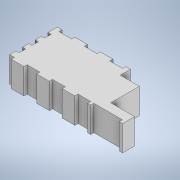
# Autodesk Inventor part: V9_BURROW_SIDE
Saved by Autodesk Inventor 2020.4 (Build 244396010, 396A)
## iProperties
Created: 2021-09-27
Part Number: V9_BURROW_SIDE
Material: Generic
Document SubType Name: Sheet Metal
Designer: YUSTE
Density: 1 g/cm^3
Sheet Metal Rule: Default
Appearance: Default
Author: YUSTE
Autodesk Inventor part; units mm, degrees
ref_plane "YZ Plane" through (0, 0, 0) normal (1, 0, 0) x (0, 1, 0)
ref_plane "XZ Plane" through (0, 0, 0) normal (0, 1, 0) x (-1, 0, 0)
ref_plane "XY Plane" through (0, 0, 0) normal (0, 0, 1) x (1, 0, 0)
sketch "Sketch1" plane through (0, 0, 0) normal (0, 1, 0) x (-1, 0, 0)
  line L0 (147.3507, -0.6443) -> (74.3257, -0.6443)
  line L1 (74.3257, -0.6443) -> (74.3257, 50.1557)
  line L2 (74.3257, 50.1557) -> (147.3507, 50.1557)
  line L3 (147.3507, 50.1557) -> (147.3507, -0.6443)
  line L4 (147.3507, 50.1557) -> (142.5882, 50.1557)
  line L5 (142.5882, 50.1557) -> (142.5882, 46.9807)
  line L6 (142.5882, 46.9807) -> (147.3507, 46.9807)
  line L7 (147.3507, 46.9807) -> (147.3507, 50.1557)
  line L8 (129.8882, 50.1557) -> (117.1882, 50.1557)
  line L9 (117.1882, 50.1557) -> (117.1882, 46.9807)
  line L10 (117.1882, 46.9807) -> (129.8882, 46.9807)
  line L11 (129.8882, 46.9807) -> (129.8882, 50.1557)
  line L12 (104.4882, 50.1557) -> (91.7882, 50.1557)
  line L13 (91.7882, 50.1557) -> (91.7882, 46.9807)
  line L14 (91.7882, 46.9807) -> (104.4882, 46.9807)
  line L15 (104.4882, 46.9807) -> (104.4882, 50.1557)
  line L16 (147.3507, 2.5307) -> (147.3507, -0.6443)
  line L17 (129.8882, -0.6443) -> (117.1882, -0.6443)
  line L18 (104.4882, -0.6443) -> (91.7882, -0.6443)
  line L19 (147.3507, 8.8807) -> (147.3507, 15.2307)
  line L20 (147.3507, 15.2307) -> (144.1757, 15.2307)
  line L21 (144.1757, 15.2307) -> (144.1757, 8.8807)
  line L22 (144.1757, 8.8807) -> (147.3507, 8.8807)
  line L23 (147.3507, 21.5807) -> (147.3507, 27.9307)
  line L24 (147.3507, 27.9307) -> (144.1757, 27.9307)
  line L25 (144.1757, 27.9307) -> (144.1757, 21.5807)
  line L26 (144.1757, 21.5807) -> (147.3507, 21.5807)
  line L27 (147.3507, 34.2807) -> (147.3507, 40.6307)
  line L28 (147.3507, 40.6307) -> (144.1757, 40.6307)
  line L29 (144.1757, 40.6307) -> (144.1757, 34.2807)
  line L30 (144.1757, 34.2807) -> (147.3507, 34.2807)
  line L31 (74.3257, 46.9807) -> (74.3257, 50.1557)
  line L32 (74.3257, 2.5307) -> (74.3257, -0.6443)
  line L33 (79.0882, -0.6443) -> (79.0882, 2.5307)
  line L34 (79.0882, 2.5307) -> (91.7882, 2.5307)
  line L35 (91.7882, 2.5307) -> (91.7882, -0.6443)
  line L36 (91.7882, -0.6443) -> (79.0882, -0.6443)
  line L37 (104.4882, 2.5307) -> (104.4882, -0.6443)
  line L38 (104.4882, -0.6443) -> (117.1882, -0.6443)
  line L39 (117.1882, -0.6443) -> (117.1882, 2.5307)
  line L40 (117.1882, 2.5307) -> (104.4882, 2.5307)
  line L41 (129.8882, -0.6443) -> (129.8882, 2.5307)
  line L42 (129.8882, 2.5307) -> (142.5882, 2.5307)
  line L43 (142.5882, 2.5307) -> (142.5882, -0.6443)
  line L44 (142.5882, -0.6443) -> (129.8882, -0.6443)
  line L45 (74.3257, 50.1557) -> (74.3257, 18.4057)
  line L46 (74.3257, 46.9807) -> (74.3257, 50.1557)
  line L47 (79.0882, 50.1557) -> (66.3882, 50.1557)
  line L48 (66.3882, 50.1557) -> (66.3882, 46.9807)
  line L49 (66.3882, 46.9807) -> (79.0882, 46.9807)
  line L50 (79.0882, 46.9807) -> (79.0882, 50.1557)
  line L51 (66.3882, 50.1557) -> (63.2132, 50.1557)
  line L52 (63.2132, 50.1557) -> (63.2132, 46.9807)
  line L53 (63.2132, 46.9807) -> (66.3882, 46.9807)
  line L54 (66.3882, 46.9807) -> (66.3882, 50.1557)
  line L55 (63.2132, 50.1557) -> (31.4632, 50.1557)
  line L56 (31.4632, 50.1557) -> (31.4632, 38.1669)
  line L57 (31.4632, 38.1669) -> (63.2132, 38.1669)
  line L58 (63.2132, 38.1669) -> (63.2132, 50.1557)
  line L59 (63.2132, 46.9807) -> (63.2132, 50.1557)
  line L60 (63.2132, 50.1557) -> (31.4632, 50.1557)
  line L61 (31.4632, 50.1557) -> (31.4632, 46.9807)
  line L62 (31.4632, 46.9807) -> (63.2132, 46.9807)
  line L63 (31.4632, 50.1557) -> (34.6382, 50.1557)
  line L64 (34.6382, 50.1557) -> (34.6382, 46.9807)
  line L65 (34.6382, 46.9807) -> (31.4632, 46.9807)
  line L66 (31.4632, 46.9807) -> (31.4632, 50.1557)
  line L67 (74.3257, 46.9807) -> (55.2757, 46.9807)
  line L68 (55.2757, 46.9807) -> (55.2757, 9.5919)
  line L69 (55.2757, 9.5919) -> (74.3257, 9.5919)
  line L70 (74.3257, 9.5919) -> (74.3257, 46.9807)
  point P0 (0, 0)
  point P1 (79.0882, -0.6443)
  point P2 (91.7882, -0.6443)
  point P3 (104.4882, -0.6443)
  point P4 (117.1882, -0.6443)
  point P5 (129.8882, -0.6443)
  point P6 (142.5882, -0.6443)
  point P7 (55.2757, 38.1669)
  dimension "d103" = 73.025
  dimension "d105" = 4.7625
  dimension "d106" = 3.175
  dimension "d107" = 12.7
  dimension "d108" = 3.175
  dimension "d109" = 12.7
  dimension "d110" = 3.175
  dimension "d111" = 12.7
  dimension "d112" = 12.7
  dimension "d121" = 6.35
  dimension "d122" = 3.175
  dimension "d123" = 6.35
  dimension "d124" = 3.175
  dimension "d126" = 6.35
  dimension "d127" = 6.35
  dimension "d128" = 3.175
  dimension "d129" = 6.35
  dimension "d146" = 3.175
  dimension "d147" = 12.7
  dimension "d148" = 0
  dimension "d149" = 4.7625
  dimension "d150" = 3.175
  dimension "d151" = 12.7
  dimension "d152" = 12.7
  dimension "d153" = 0
  dimension "d154" = 3.175
  dimension "d155" = 12.7
  dimension "d156" = 12.7
  dimension "d161" = 0
  dimension "d168" = 12.7
  dimension "d169" = 3.175
  dimension "d170" = 12.7
  dimension "d171" = 3.175
  dimension "d172" = 3.175
  dimension "d182" = 31.75
  dimension "d183" = 11.9888
  dimension "d186" = 3.175
  dimension "d195" = 19.05
  dimension "d196" = 37.3888
  constraints: 140 end point, 32 parallel, 18 perpendicular, 13 point on line, 2 horizontal, 2 vertical, 1 collinear, 11 other
  measures "d103" distance of L0.start L0.end
  measures "d105" distance of L3.start L4.end
  measures "d106" distance of L5.end L4.end
  measures "d107" distance of L8.start L8.end
  measures "d108" distance of L9.end L8.end
  measures "d109" distance of L12.start L12.end
  measures "d110" distance of L13.end L12.end
  measures "d111" distance between parallel lines of L5 L11
  measures "d112" distance between parallel lines of L15 L9
  measures "d121" distance of L19.start L19.end
  measures "d122" distance of L20.end L19.end
  measures "d123" distance of L23.start L23.end
  measures "d124" distance of L24.end L23.end
  measures "d126" distance between parallel lines of L26 L20
  measures "d127" distance of L27.start L27.end
  measures "d128" distance of L28.end L27.end
  measures "d129" distance between parallel lines of L24 L30
  measures "d146" distance of L33.start L33.end
  measures "d147" distance of L33.end L34.end
  measures "d148" distance between parallel lines of L0 L36
  measures "d149" distance between parallel lines of L1 L33
  measures "d150" distance of L37.start L37.end
  measures "d151" distance of L38.end L37.end
  measures "d152" distance between parallel lines of L35 L37
  measures "d153" distance between parallel lines of L0 L38
  measures "d154" distance of L41.start L41.end
  measures "d155" distance of L41.end L42.end
  measures "d156" distance between parallel lines of L39 L41
  measures "d161" distance between parallel lines of L1 L45
  measures "d168" distance of L47.start L47.end
  measures "d169" distance of L48.end L47.end
  measures "d170" distance between parallel lines of L13 L50
  measures "d171" distance of L47.end L51.end
  measures "d172" distance of L52.end L51.end
  measures "d182" distance of L51.end L55.end
  measures "d183" distance of L56.end L55.end
  measures "d186" distance of L60.end L63.end
  measures "d195" distance of L46.start L67.end
  measures "d196" distance of L68.end L67.end
extrude "Extrusion15" add sketch "Sketch1" along normal blind 25.4 contours L0 L43 L42 L41 L39 L40 L37 L35 L34 L33 L1 L49 L50 L2 L13 L14 L15 L9 L10 L11 L5 L6 L3 L28 L29 L30 L24 L25 L26 L20 L21 L22 | L69 L68 L57 L58 L53 L49 L1 | L68 L62 L58 L57 | L57 L56 L62 L68 | L53 L52 L51 L48 | L56 L55 L64 L62
equation "\"BendRadius\" = Thickness"
equation "\"BendReliefWidth\" = Thickness"
equation "\"BendReliefDepth\" = 0.5 * Thickness"
equation "\"CornerReliefSize\" = 4 * Thickness"
equation "\"MinimumRemnant\" = 2 * Thickness"
equation "\"TransitionRadius\" = BendRadius"
equation "\"JacobiRadiusSize\" = BendRadius"
equation "\"GapSize\" = Thickness"
equation "\"Thickness\" = 3.048"
body "Solid17"
